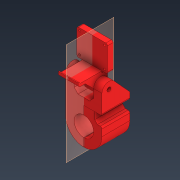
# Autodesk Inventor part: CH_01_0047_camera_mount
Saved by Autodesk Inventor 2022.3 (Build 263350030, 350C)
## iProperties
Created: 2022-08-15
Part Number: CH_01_0047_camera_mount
Material: Generic
Document SubType Name: Modeling
Designer: Tomasz Krakowski
Density: 1 g/cm^3
Appearance: Light Red-Orange
Author: Tomasz Krakowski
Autodesk Inventor part; units mm, degrees
ref_plane "XZ Plane" through (0, 0, 0) normal (0, 1, 0) x (-1, 0, 0)
ref_plane "XY Plane" through (0, 0, 0) normal (0, 0, 1) x (1, 0, 0)
sketch "Sketch1" plane through (0, 0, 0) normal (0, 0, 1) x (1, 0, 0)
  arc A0 (1, -17.4714) -> (0, -17.5) centre (0, 0) ccw
  line L0 (1, -32.4846) -> (1, -17.4714)
  line L1 (-32.5, 0) -> (-32.5, 80)
  line L2 (32.5, 80) -> (32.5, 0)
  line L3 (-17.5, 80) -> (-17.5, 45)
  line L4 (-17.5, 45) -> (17.5, 45)
  line L5 (17.5, 45) -> (17.5, 80)
  line L6 (-32.5, 80) -> (-17.5, 80)
  line L7 (17.5, 80) -> (32.5, 80)
  line L8 (0, -17.5) -> (0, -32.5)
  line L9 (0, -17.5) -> (0, 0) construction
  arc A1 (1, -32.4846) -> (32.5, 0) centre (0, 0) ccw
  arc A2 (-32.5, 0) -> (0, -32.5) centre (0, 0) ccw
  line L10 (0, 17.5) -> (0, 32.5)
  line L11 (0, 32.5) -> (32.5, 32.5)
  line L12 (0, 0) -> (0, 17.5) construction
  line L13 (32.5, 15) -> (19.5, 15)
  line L14 (19.5, 15) -> (19.5, 32.5)
  dimension "d0" = 35
  dimension "d2" = 45
  dimension "d3" = 35
  dimension "d4" = 35
  dimension "d5" = 1
  dimension "d6" = 65
  dimension "d7" = 32.5
  dimension "d9" = 15
  dimension "d43" = 17.5
  dimension "d44" = 13
  constraints: 30 end point, 9 perpendicular, 7 point on circle, 5 vertical, 4 collinear, 3 centre point, 3 coincident, 3 point on line, 2 tangent, 1 horizontal
  measures "d0" diameter of A0
  measures "d2" distance from line of point (0, 0) L4
  measures "d3" distance between parallel lines of L5 L3
  measures "d4" distance between parallel lines of L4 L6
  measures "d5" distance between parallel lines of L0 L8
  measures "d6" distance between parallel lines of L2 L1
  measures "d7" radius of A2
  measures "d9" distance of L10.start L10.end
  measures "d43" distance of L13.end L14.end
  measures "d44" distance between parallel lines of L2 L14
extrude "Extrusion1" add sketch "Sketch1" along normal blind 50 contours A0 L8 A2 L1 L6 L3 L4 L5 L7 L2 L11 L10
sketch "Sketch2" plane through (0, 17.5, 0) normal (1, 0, 0) x (0, 0, -1)
  line L0 (-50, 0) -> (-50, 15) construction
  line L1 (-50, 7.5) -> (0, 7.5) construction
  line L2 (0, 62.5) -> (0, -17.5) construction
  line L3 (-50, -50) -> (-50, -35) construction
  line L4 (-50, -42.5) -> (0, -42.5) construction
  line L5 (-37.5, -42.5) -> (-37.5, 7.5) construction
  line L6 (-12.5, -42.5) -> (-12.5, 7.5) construction
  dimension "d12" = 12.5
  dimension "d13" = 12.5
  constraints: 8 end point, 5 point on line, 2 horizontal, 2 midpoint, 2 vertical
  measures "d12" distance of L5.end L1.start
  measures "d13" distance of L1.end L6.end
hole "Hole1" at (0, 25, 37.5) at (0, 25, 12.5) at (0, -25, 37.5) at (0, -25, 12.5) direction (-1, 0, 0) diameter 5.5 depth 12
sketch "Sketch3" plane through (32.5, 32.5, 0) normal (1, 0, 0) x (0, 0, -1)
  line L0 (0, 12.5) -> (-28.2734, 43.4332)
  arc A0 (-28.2734, 43.4332) -> (-50, 35) centre (-37.5, 35) ccw
  line L1 (-50, 0) -> (-50, 47.5) projected
  line L2 (-50, 35) -> (-50, 47.5) construction
  line L3 (-50, 47.5) -> (-37.5, 47.5)
  line L4 (0, 0) -> (0, 47.5) construction
  line L5 (-37.5, 47.5) -> (0, 47.5)
  line L6 (0, 47.5) -> (-50, 47.5) construction
  line L7 (-50, 35) -> (-50, 47.5) construction
  line L8 (-50, 35) -> (-50, 47.5) construction
  line L9 (-50, 47.5) -> (-37.5, 47.5) construction
  line L10 (-37.5, 47.5) -> (0, 47.5) construction
  line L11 (0, 47.5) -> (0, 12.5)
  point P0 (0, -32.5)
  dimension "d22" = 25
  constraints: 18 end point, 5 tangent, 3 collinear, 3 point on circle, 2 perpendicular, 1 centre point, 1 point on line
  measures "d22" diameter of A0
extrude "Extrusion2" cut sketch "Sketch3" against normal through all
chamfer "Chamfer1" distance 7 angle 45 2 edges at (17.5, 45, 25) (-17.5, 45, 25)
sketch "Sketch4" plane through (32.5, 32.5, 50) normal (1, 0, 0) x (0, 0, -1)
  arc A0 (21.7266, 43.4332) -> (0, 35) centre (12.5, 35) ccw construction
  point P0 (50, -32.5)
  constraints: 1 coincident
hole "Hole2" at (32.5, 67.5, 37.5) direction (-1, 0, 0) diameter 4.5 depth 15 counterbore diameter 7.1 counterbore depth 4.1
sketch "Sketch5" plane through (-17.5, 52, 50) normal (1, 0, 0) x (0, 0, -1)
  circle A0 centre (12.5, 15.5) radius 2.25 projected
  circle A1 centre (12.5, 15.5) radius 2.25 projected
  point P0 (50, -52)
  constraints: 1 coincident
hole "Hole3" at (-17.5, 67.5, 37.5) direction (-1, 0, 0) diameter 5.5 depth 15
extrude "Extrusion3" add sketch "Sketch1" along normal up to surface (50 mm away) separate body contours A0 L10 L11 L14 L13 L2 A1 L0
sketch "Sketch6" plane through (19.5, 15, 0) normal (1, 0, 0) x (0, 0, -1)
  circle A0 centre (-37.5, 10) radius 2.75 projected
  circle A1 centre (-12.5, 10) radius 2.75 projected
  circle A2 centre (-37.5, -40) radius 2.75 projected
  circle A3 centre (-12.5, -40) radius 2.75 projected
  circle A4 centre (-37.5, -40) radius 2.75 projected
  point P0 (0, -15)
  point P1 (-37.5, 10)
  point P2 (-12.5, 10)
  constraints: 4 coincident
hole "Hole4" at (19.5, 25, 12.5) at (19.5, 25, 37.5) at (19.5, -25, 37.5) at (19.5, -25, 12.5) direction (-1, 0, 0) diameter 4.5 end through all start extended yes counterbore diameter 7.1 counterbore depth 4.1 bodies 2
chamfer "Chamfer2" distance 5 angle 45 1 edges at (19.5, 15, 25)
fillet "Fillet2" radius 3 2 edges at (32.5, 32.5, 25) (32.5, 15, 25)
sketch "Sketch7" plane through (0, 0, 0) normal (1, 0, 0) x (0, 1, 0)
  circle A0 centre (67.5, 37.5) radius 2.75 projected
  circle A1 centre (67.5, 37.5) radius 2
  circle A2 centre (67.5, 37.5) radius 12.5
  line L0 (67.5, 50) -> (87.5, 50)
  line L1 (87.5, 50) -> (87.5, 35)
  line L2 (87.5, 35) -> (134.5, 35)
  line L3 (52, 6.3981) -> (52, 50) projected
  line L4 (134.5, 35) -> (134.5, 25)
  line L5 (134.5, 25) -> (67.5, 25)
  point P0 (0, 0)
  dimension "d58" = 4
  dimension "d59" = 25
  dimension "d60" = 20
  dimension "d61" = 10
  dimension "d62" = 47
  constraints: 10 end point, 3 perpendicular, 2 centre point, 2 coincident, 2 point on circle, 2 tangent, 1 horizontal, 1 parallel
  measures "d58" diameter of A1
  measures "d59" diameter of A2
  measures "d60" distance from line of A1.centre L1
  measures "d61" distance from line of L5 L1.end
  measures "d62" distance between parallel lines of L1 L4
extrude "Extrusion4" add sketch "Sketch7" along normal mid plane 35 separate body contours A2 | A2 L0 L1 L2 L4 L5
sketch "Sketch8" plane through (17.5, 134.5, 25) normal (0, 0, -1) x (-1, 0, 0)
  line L0 (45, -47) -> (-10, -47)
  line L1 (-10, -47) -> (-10, 0)
  line L2 (-10, 0) -> (45, 0)
  line L3 (45, 0) -> (45, -47)
  line L4 (45, -47) -> (-10, 0) construction
  line L5 (-10, -47) -> (45, 0) construction
  line L6 (17.5, -134.5) -> (17.5, -23.5) construction
  line L7 (35, -47) -> (0, -47) construction
  point P0 (0, 0)
  dimension "d65" = 55
  constraints: 14 end point, 2 midpoint, 2 parallel, 1 collinear, 1 horizontal, 1 perpendicular, 1 point on line, 1 vertical
  measures "d65" distance between parallel lines of L3 L1
extrude "Extrusion5" add sketch "Sketch8" against normal up to surface (10 mm away) bodies 3
fillet "Fillet3" radius 3 6 edges at (27.5, 134.5, 30) (-27.5, 134.5, 30) (-17.5, 87.5, 30) (-27.5, 87.5, 30) (17.5, 87.5, 30) (27.5, 87.5, 30)
sketch "Sketch9" plane through (17.5, 67.5, 25) normal (0, 0, -1) x (-1, 0, 0)
  line L0 (-5, 25) -> (40, 25) construction
  line L1 (40, 25) -> (40, 62.5) construction
  line L2 (40, 62.5) -> (-5, 62.5) construction
  line L3 (-5, 62.5) -> (-5, 25) construction
  line L4 (-5, 25) -> (40, 62.5) construction
  line L5 (40, 25) -> (-5, 62.5) construction
  line L6 (17.5, 43.75) -> (17.5, 67) construction
  line L7 (42, 67) -> (-7, 67) construction
  line L8 (-7, 20) -> (-3, 20) projected
  point P0 (17.5, -67.5)
  dimension "d69" = 45
  dimension "d70" = 37.5
  dimension "d79" = 5
  constraints: 14 end point, 3 midpoint, 2 parallel, 2 perpendicular, 1 horizontal
  measures "d69" distance of L1.end L2.end
  measures "d70" distance between parallel lines of L2 L0
  measures "d79" distance between parallel lines of L0 L8
hole "Hole5" at (22.5, 92.5, 25) at (22.5, 130, 25) at (-22.5, 130, 25) at (-22.5, 92.5, 25) direction (0, 0, 1) diameter 3.5 end through all start extended yes counterbore diameter 5.5 counterbore depth 3 bodies 3
sketch "Sketch10" plane through (-17.5, 67.5, 50) normal (0, 0, 1) x (1, 0, 0)
  line L0 (0, 20) -> (35, 20) projected
  line L1 (0, 20) -> (35, 20)
  line L2 (35, 20) -> (35, 15)
  line L3 (35, 15) -> (0, 15)
  line L4 (0, 15) -> (0, 20)
  line L5 (35, 20) -> (35, 0) construction
  point P0 (17.5, -67.5)
  dimension "d80" = 5
  constraints: 8 end point, 2 parallel, 1 collinear, 1 horizontal, 1 perpendicular
  measures "d80" distance between parallel lines of L0 L3
extrude "Extrusion6" add sketch "Sketch10" along normal blind 28 bodies 3
sketch "Sketch11" plane through (17.5, 0, 0) normal (1, 0, 0) x (0, 0, -1)
  line L0 (-50, 67.5) -> (-50, 0) projected
  line L1 (-50, 67.5) -> (-65, 82.5)
  line L2 (-50, 82.5) -> (-78, 82.5) construction
  line L3 (-50, 67.5) -> (-50, 82.5)
  arc A0 (-28.2734, 75.9332) -> (-50, 67.5) centre (-37.5, 67.5) ccw projected
  line L4 (-50, 82.5) -> (-50, 67.5) projected
  line L5 (-50, 82.5) -> (-65, 82.5)
  point P0 (0, 0)
  dimension "d83" = 15
  constraints: 6 end point, 1 perpendicular, 1 point on line, 1 tangent, 1 vertical
  measures "d83" distance of L1.end L2.start
extrude "Extrusion7" add sketch "Sketch11" against normal blind 5 bodies 3
mirror "Mirror1" about plane through (0, 0, 0) normal (1, 0, 0) of "Extrusion7" bodies 3
sketch "Sketch12" plane through (-17.5, 87.5, 35) normal (0, 1, 0) x (1, 0, 0)
  line L0 (0, -43) -> (35, -43) projected
  line L1 (35, -30) -> (35, -43) construction
  line L2 (0, -43) -> (35, -43)
  line L3 (35, -43) -> (35, -38.5)
  line L4 (35, -38.5) -> (0, -38.5)
  line L5 (0, -38.5) -> (0, -43)
  line L6 (-7, 0) -> (42, 0) projected
  point P0 (17.5, 35)
  dimension "d86" = 38.5
  constraints: 8 end point, 2 parallel, 1 horizontal, 1 perpendicular, 1 point on line
  measures "d86" distance between parallel lines of L6 L4
extrude "Extrusion8" add sketch "Sketch12" along normal blind 3 bodies 3
chamfer "Chamfer3" distance 3 angle 45 3 edges at (0, 90.5, 73.5) (0, 82.5, 78) (0, 82.5, 50)
equation "\"d13\" = d12"
body "Solid1"
body "Solid2"
body "Solid3"
